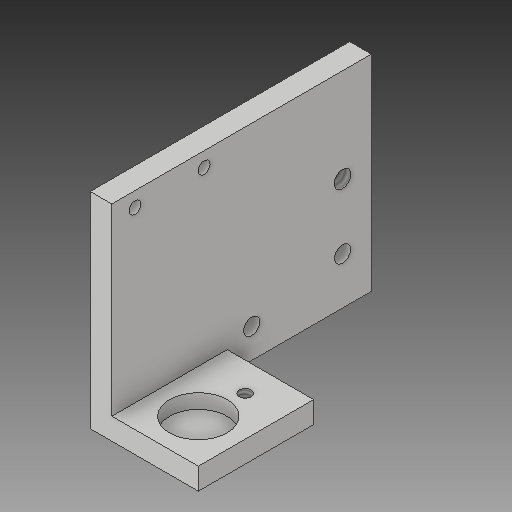
# Autodesk Inventor part: WheelIntake4.0Base
Saved by Autodesk Inventor 2017 (Build 210142000, 142)
## iProperties
Created: 2017-12-13
Part Number: WheelIntake4.0Base
Material: Generic
Document SubType Name: Modeling
Designer: User
Density: 1 g/cm^3
Appearance: Default
Mass: 15.5086 g
Surface Area: 81.5416 cm^2
Volume: 15.5086 cm^3
Author: User
Autodesk Inventor part; units mm, degrees
ref_plane "YZ Plane" through (0, 0, 0) normal (1, 0, 0) x (0, 1, 0)
ref_plane "XZ Plane" through (0, 0, 0) normal (0, 1, 0) x (-1, 0, 0)
ref_plane "XY Plane" through (0, 0, 0) normal (0, 0, 1) x (1, 0, 0)
sketch "Sketch1" plane through (0, 0, 0) normal (1, 0, 0) x (0, 1, 0)
  line L0 (0, 0) -> (45.2437, 0)
  line L1 (45.2437, 0) -> (45.2438, -57.15)
  line L2 (45.2438, -57.15) -> (0, -57.15)
  line L3 (0, -57.15) -> (0, 0)
  dimension "d0" = 45.2437
  dimension "d1" = 57.15
  constraints: 8 end point, 2 parallel, 1 horizontal, 1 perpendicular
  measures "d0" distance of L1.end L2.end
  measures "d1" distance of L0.end L1.end
extrude "Extrusion1" add sketch "Sketch1" along normal blind 4.7625
sketch "Sketch3" plane through (4.7625, 0, 0) normal (1, 0, 0) x (0, 0, -1)
  line L0 (0, 45.2437) -> (0, 0) projected
  line L1 (0, 0) -> (57.15, 0) projected
  line L2 (57.15, 0) -> (57.15, 45.2438) projected
  line L3 (57.15, 45.2438) -> (0, 45.2437) projected
  line L4 (0, 0) -> (25.4, 0)
  line L5 (25.4, 0) -> (25.4, 4.7625)
  line L6 (25.4, 4.7625) -> (0, 4.7625)
  line L7 (0, 4.7625) -> (0, 0)
  dimension "d8" = 4.7625
  constraints: 8 end point, 2 parallel, 1 horizontal, 1 perpendicular
  measures "d8" distance of L5.end L4.end
extrude "Extrusion3" add sketch "Sketch3" along normal blind 19.05 contours L6 L5 L1 L0
sketch "Sketch4" plane through (0, 0, 0) normal (-1, 0, 0) x (0, 0, 1)
  line L0 (0, 0) -> (0, 45.2437) projected
  line L1 (0, 45.2437) -> (-57.15, 45.2438) projected
  line L2 (-57.15, 45.2438) -> (-57.15, 0) projected
  line L3 (-57.15, 0) -> (0, 0) projected
  line L4 (-57.15, 45.2438) -> (0, 45.2437) projected
  line L5 (-57.15, 45.2438) -> (-44.45, 45.2438)
  line L6 (-57.15, 29.3688) -> (-57.15, 45.2438)
  line L7 (-57.15, 0) -> (-57.15, 45.2438) projected
  line L8 (-57.15, 32.5438) -> (-44.45, 32.5438)
  line L9 (-44.45, 32.5438) -> (-44.45, 16.6688)
  line L10 (-44.45, 16.6688) -> (-57.15, 16.6688)
  line L11 (-57.15, 16.6688) -> (-57.15, 32.5438)
  point P0 (-12.7, 45.2437)
  dimension "d48" = 15.875
  dimension "d49" = 12.7
  dimension "d50" = 12.7
  constraints: 12 end point, 2 horizontal, 2 parallel, 1 perpendicular, 1 point on line
  measures "d48" distance of L8.end L9.end
  measures "d49" distance between parallel lines of L1 L8
  measures "d50" distance of L8.start L8.end
extrude "Extrusion4" add sketch "Sketch4" along normal blind 7.9375 contours L2 L8 L9 L10
sketch "Sketch5" plane through (4.7625, 0, 0) normal (1, 0, 0) x (0, 0, -1)
  line L0 (25.4, 4.7625) -> (25.4, 0) projected
  line L1 (25.4, 0) -> (57.15, 0) projected
  line L2 (57.15, 0) -> (57.15, 45.2438) projected
  line L3 (57.15, 45.2438) -> (0, 45.2437) projected
  line L4 (0, 45.2437) -> (0, 4.7625) projected
  line L5 (0, 4.7625) -> (25.4, 4.7625) projected
  line L6 (0, 45.2437) -> (0, 40.4812) projected
  line L7 (0, 40.4812) -> (12.7, 40.4812) projected
  line L8 (12.7, 40.4812) -> (12.7, 45.2437) projected
  line L9 (12.7, 45.2437) -> (0, 45.2437) projected
  point P0 (0, 0)
  point P1 (50.8, 24.6063)
  dimension "d16" = 20.6375
  dimension "d17" = 6.35
  measures "d16" distance from line of L3 point (50.8, 24.606)
  measures "d17" distance from line of L2 point (50.8, 24.606)
hole "Hole1" at (4.7625, 24.6063, -50.8) direction (-1, 0, 0) diameter 3.683 depth 14.9352 tip angle 118 thread size "10-24 UNC" class "2B" standard "ANSI Unified Screw Threads"
sketch "Sketch6" plane through (4.7625, 4.7625, 0) normal (0, 1, 0) x (1, 0, 0)
  line L0 (0, 0) -> (0, 25.4) projected
  line L1 (0, 0) -> (19.05, 0) projected
  line L2 (19.05, 25.4) -> (19.05, 0) projected
  line L3 (0, 25.4) -> (19.05, 25.4) projected
  point P0 (-4.7625, 0)
  point P1 (9.525, 9.525)
  dimension "d25" = 9.525
  dimension "d26" = 9.525
  measures "d25" distance from line of L0 point (9.525, 9.525)
  measures "d26" distance from line of L1 point (9.525, 9.525)
hole "Hole2" at (14.2875, 4.7625, -9.525) direction (0, -1, 0) diameter 12.7 depth 3.175
sketch "Sketch10" plane through (0, 45.2438, 0) normal (0, 1, 0) x (1, 0, 0)
  line L0 (0, 0) -> (0, 57.15) projected
  line L1 (0, 0) -> (4.7625, 0) projected
  line L2 (4.7625, 57.15) -> (4.7625, 0) projected
  line L3 (0, 57.15) -> (4.7625, 57.15) projected
  point P0 (0, 0)
  point P1 (11.1125, 6.35)
hole "Hole3" at (11.1125, 45.2438, -6.35) direction (0, -1, 0) diameter 2.6416 depth 10.9728 tip angle 118 thread size "6-32 UNC" class "2B" standard "ANSI Unified Screw Threads"
sketch "Sketch11" plane through (0, 0, -57.15) normal (0, -1, 0) x (1, 0, 0)
  line L0 (0, 0) -> (0, 57.15) projected
  line L1 (0, 0) -> (4.7625, 0) projected
  line L2 (4.7625, 31.75) -> (4.7625, 0) projected
  line L3 (4.7625, 31.75) -> (23.8125, 31.75) projected
  line L4 (23.8125, 57.15) -> (23.8125, 31.75) projected
  line L5 (0, 57.15) -> (23.8125, 57.15) projected
  point P0 (15.0812, 38.1)
  dimension "d58" = 6.35
  measures "d58" distance from line of L3 point (15.081, 38.1)
hole "Hole4" at (15.0812, 0, -19.05) direction (0, 1, 0) diameter 2.6416 end through all thread size "6-32 UNC" class "2B" standard "ANSI Unified Screw Threads"
sketch "Sketch12" plane through (4.7625, 0, 0) normal (1, 0, 0) x (0, 0, -1)
  circle A0 centre (50.8, 24.6063) radius 1.8415 projected
  line L0 (25.4, 4.7625) -> (25.4, 0) projected
  line L1 (25.4, 0) -> (57.15, 0) projected
  line L2 (57.15, 0) -> (57.15, 45.2438) projected
  line L3 (57.15, 45.2438) -> (0, 45.2437) projected
  line L4 (0, 45.2437) -> (0, 4.7625) projected
  line L5 (0, 4.7625) -> (25.4, 4.7625) projected
  point P0 (0, 0)
  point P1 (50.8, 10.3124)
  point P2 (30.7975, 6.5024)
  dimension "d66" = 6.35
  dimension "d67" = 10.3124
  dimension "d68" = 6.5024
  dimension "d69" = 26.3525
  measures "d66" distance from line of L2 point (50.8, 10.312)
  measures "d67" distance from line of L1 point (50.8, 10.312)
  measures "d68" distance from line of L1 point (30.797, 6.502)
  measures "d69" distance from line of L2 point (30.797, 6.502)
hole "Hole5" at (4.7625, 10.3124, -50.8) at (4.7625, 6.5024, -30.7975) direction (-1, 0, 0) diameter 3.556 end through all
sketch "Sketch13" plane through (4.7625, 0, 0) normal (1, 0, 0) x (0, 0, -1)
  line L0 (0, 45.2437) -> (0, 4.7625) projected
  point P0 (0, 0)
  point P1 (5.08, 42.0254)
  point P2 (20.32, 42.0254)
  dimension "d77" = 5.08
  dimension "d78" = 15.24
  measures "d77" distance from line of point (5.08, 42.025) L0
  measures "d78" distance of point (5.08, 42.025) point (20.32, 42.025)
hole "Hole6" at (4.7625, 42.0254, -5.08) at (4.7625, 42.0254, -20.32) direction (-1, 0, 0) diameter 2.6416 end through all
body "Solid1"
